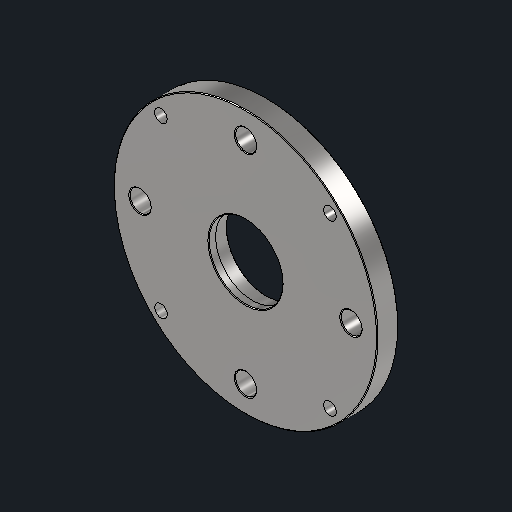
# Autodesk Inventor part: VF65-KF40-adapter
Saved by Autodesk Inventor 2026 (Build 300175050, 175E)
## iProperties
Created: 2026-02-02
Part Number: VF65-KF40-adapter
Material: Stainless Steel
Document SubType Name: Modeling
Designer: queezz
Density: 8 g/cm^3
Appearance: Semi-Polished
Author: queezz
Autodesk Inventor part; units mm, degrees
ref_plane "YZ Plane" through (0, 0, 0) normal (1, 0, 0) x (0, 1, 0)
ref_plane "XZ Plane" through (0, 0, 0) normal (0, 1, 0) x (-1, 0, 0)
ref_plane "XY Plane" through (0, 0, 0) normal (0, 0, 1) x (1, 0, 0)
sketch "Sketch1" plane through (0, 0, 0) normal (0, 0, 1) x (1, 0, 0)
  circle A0 centre (0, 0) radius 75
  dimension "d0" = 150
  constraints: 1 centre point, 1 coincident
  measures "d0" diameter of A0
extrude "Extrusion1" add sketch "Sketch1" along normal blind 12
sketch "Sketch2" plane through (0, 0, 12) normal (0, 0, 1) x (1, 0, 0)
  circle A0 centre (0, 0) radius 60 construction
  point P0 (60, 0)
  dimension "d3" = 120
  constraints: 2 horizontal alignment, 1 coincident, 2 other
hole "Hole1" at (60, 0, 12) direction (0, 0, -1) diameter 12 end through all
pattern_circular "Circular Pattern1" count 4 over 360 about axis through (0, 0, 0) along (0, 0, 1) of "Hole1"
sketch "Sketch3" plane through (0, 0, 12) normal (0, 0, 1) x (1, 0, 0)
  circle A0 centre (0, 0) radius 68 construction
  line L0 (48.0833, 48.0833) -> (0, 0) construction
  line L1 (0, 0) -> (75, 0) construction
  circle A1 centre (0, 0) radius 75 projected
  dimension "d14" = 136
  dimension "d15" = 45
  constraints: 4 end point, 1 coincident, 1 horizontal, 1 horizontal alignment, 4 other
  measures "d15" angle of L1 L0
hole "Hole2" at (48.0833, 48.0833, 12) direction (0, 0, -1) diameter 7.2 end through all
pattern_circular "Circular Pattern2" count 4 over 360 about axis through (0, 0, 0) along (0, 0, 1) of "Hole2"
sketch "Sketch4" plane through (0, 0, 0) normal (1, 0, 0) x (0, 1, 0)
  line L0 (0, 0) -> (0, 12)
  line L1 (75, 12) -> (-75, 12) projected
  line L2 (75, 0) -> (-75, 0) projected
  line L3 (22.5, 0) -> (22.5, 8)
  line L4 (22.5, 8) -> (21, 8)
  line L5 (21, 8) -> (21, 12)
  dimension "d26" = 45
  dimension "d27" = 4
  dimension "d28" = 42
  constraints: 8 end point, 3 perpendicular, 2 point on line, 1 midpoint
  measures "d26" diameter of L3 L0
  measures "d27" distance of L4.end L5.end
  measures "d28" diameter of L5 L0
revolve "Revolution1" cut sketch "Sketch4" angle 360 about axis through (0, 0, 0) along (0, 0, 1)
chamfer "Chamfer1" distance 0.4 angle 45 4 edges at (-75, 0, 0) (-75, 0, 12) (0, -21, 12) (0, -22.5, 0)
chamfer "Chamfer2" distance 0.4 angle 45 8 edges at (-6, 60, 12) (-60, -6, 12) (6, -60, 12) (60, 6, 12) (-6, 60, 0) (-60, -6, 0) (60, 6, 0) (6, -60, 0)
body "Solid1"
